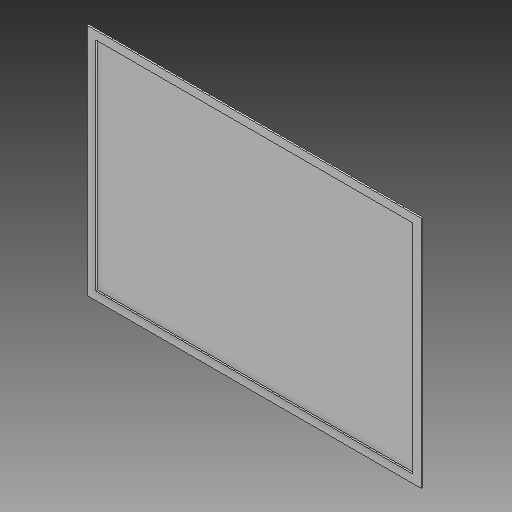
# Autodesk Inventor part: Deckel
Saved by Autodesk Inventor 2021 (Build 250183000, 183)
## iProperties
Created: 2021-10-18
Part Number: Deckel
Material: Generisch
Document SubType Name: Modeling
Designer: lukas
Density: 1 g/cm^3
Appearance: Vorgabe
Stock Number: Deckel Schaltkasten
Author: lukas
Autodesk Inventor part; units mm, degrees
ref_plane "YZ Plane" through (0, 0, 0) normal (1, 0, 0) x (0, 1, 0)
ref_plane "XZ Plane" through (0, 0, 0) normal (0, 1, 0) x (-1, 0, 0)
ref_plane "XY Plane" through (0, 0, 0) normal (0, 0, 1) x (1, 0, 0)
sketch "Skizze1" plane through (0, 0, 0) normal (0, 0, 1) x (1, 0, 0)
  line L0 (-273.7, 0) -> (273.7, 0) projected
  line L1 (0, -189.7) -> (0, 189.7) projected
  line L2 (-195.5, 135.5) -> (195.5, 135.5)
  line L3 (195.5, 135.5) -> (195.5, -135.5)
  line L4 (195.5, -135.5) -> (-195.5, -135.5)
  line L5 (-195.5, -135.5) -> (-195.5, 135.5)
  point P0 (0, 0)
  dimension "d0" = 391
  dimension "d1" = 271
  constraints: 8 end point, 2 parallel, 1 horizontal, 1 perpendicular, 2 other
  measures "d0" distance between parallel lines of L3 L5
  measures "d1" distance between parallel lines of L2 L4
extrude "Extrusion1" add sketch "Skizze1" against normal blind 2
sketch "Skizze2" plane through (0, 0, 0) normal (0, 0, 1) x (1, 0, 0)
  line L0 (-190.5, 130.5) -> (190.5, 130.5)
  line L1 (190.5, 130.5) -> (190.5, -130.5)
  line L2 (190.5, -130.5) -> (-190.5, -130.5)
  line L3 (-190.5, -130.5) -> (-190.5, 130.5)
  line L4 (195.5, -135.5) -> (195.5, 135.5) projected
  line L5 (195.5, 135.5) -> (-195.5, 135.5) projected
  line L6 (-195.5, 135.5) -> (-195.5, -135.5) projected
  line L7 (-195.5, -135.5) -> (195.5, -135.5) projected
  point P0 (0, 0)
  dimension "d12" = 5
  dimension "d13" = 5
  dimension "d14" = 5
  dimension "d15" = 5
  constraints: 8 end point, 2 parallel, 1 horizontal, 1 perpendicular
  measures "d12" distance between parallel lines of L4 L1
  measures "d13" distance between parallel lines of L5 L0
  measures "d14" distance between parallel lines of L6 L3
  measures "d15" distance between parallel lines of L7 L2
extrude "Extrusion2" add sketch "Skizze2" along normal blind 2
sketch "Skizze3" plane through (0, 0, 2) normal (0, 0, 1) x (1, 0, 0)
  line L0 (-200.5, 140.5) -> (200.5, 140.5)
  line L1 (200.5, 140.5) -> (200.5, -140.5)
  line L2 (200.5, -140.5) -> (-200.5, -140.5)
  line L3 (-200.5, -140.5) -> (-200.5, 140.5)
  line L4 (195.5, 135.5) -> (-195.5, 135.5) projected
  line L5 (-195.5, -135.5) -> (195.5, -135.5) projected
  line L6 (195.5, -135.5) -> (195.5, 135.5) projected
  line L7 (-195.5, 135.5) -> (-195.5, -135.5) projected
  point P0 (0, 0)
  dimension "d18" = 5
  dimension "d19" = 5
  dimension "d20" = 5
  dimension "d21" = 5
  constraints: 8 end point, 2 parallel, 1 horizontal, 1 perpendicular
  measures "d18" distance between parallel lines of L0 L4
  measures "d19" distance between parallel lines of L2 L5
  measures "d20" distance between parallel lines of L1 L6
  measures "d21" distance between parallel lines of L7 L3
extrude "Extrusion3" add sketch "Skizze3" against normal blind 2
